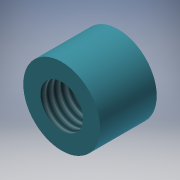
# Autodesk Inventor part: Hopper Roller Rear Plug
Saved by Autodesk Inventor 2017 (Build 210142000, 142)
## iProperties
Created: 2017-01-17
Part Number: Hopper Roller Rear Plug
Material: Generic
Document SubType Name: Modeling
Designer: Ben
Density: 1 g/cm^3
Appearance: Cadet Blue
Author: Ben
Autodesk Inventor part; units mm, degrees
ref_plane "YZ Plane" through (0, 0, 0) normal (1, 0, 0) x (0, 1, 0)
ref_plane "XZ Plane" through (0, 0, 0) normal (0, 1, 0) x (-1, 0, 0)
ref_plane "XY Plane" through (0, 0, 0) normal (0, 0, 1) x (1, 0, 0)
sketch "Sketch1" plane through (0, 0, 0) normal (0, 0, 1) x (1, 0, 0)
  circle A0 centre (0, 0) radius 9.525 construction
  circle A1 centre (0, 0) radius 8.636
  circle A2 centre (0, 0) radius 4.7625
  dimension "d0" = 19.05
  dimension "d10" = 9.525
  dimension "d13" = 17.272
  constraints: 3 centre point, 3 coincident
  measures "d0" diameter of A0
  measures "d10" diameter of A2
  measures "d13" diameter of A1
extrude "Extrusion1" add sketch "Sketch1" along normal blind 12.7
thread "Thread1" size "3/8-16 UNC" class "2B" standard "ANSI Unified Screw Threads" full length
body "Solid1"
